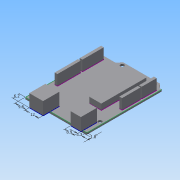
# Autodesk Inventor part: arduino_uno
Saved by Autodesk Inventor 2015 (Build 190159000, 159)
## iProperties
Created: 2016-01-04
Part Number: arduino_uno
Material: Generic
Document SubType Name: Modeling
Designer: JoshuaYuan
Density: 1 g/cm^3
Appearance: Default
Author: JoshuaYuan
Autodesk Inventor part; units mm, degrees
ref_plane "YZ Plane" through (0, 0, 0) normal (1, 0, 0) x (0, 1, 0)
ref_plane "XZ Plane" through (0, 0, 0) normal (0, 1, 0) x (-1, 0, 0)
ref_plane "XY Plane" through (0, 0, 0) normal (0, 0, 1) x (1, 0, 0)
sketch "Sketch1" plane through (0, 0, 0) normal (0, 1, 0) x (-1, 0, 0)
  line L0 (53.3, 0) -> (0, 0)
  line L1 (0, 0) -> (0, -65)
  line L2 (0, -65) -> (2, -65)
  line L3 (2, -65) -> (5, -68.6)
  line L4 (5, -68.6) -> (37, -68.6)
  line L5 (37, -68.6) -> (40, -65)
  line L6 (40, -65) -> (52.46, -65)
  line L7 (52.46, -65) -> (53.3, -64.3)
  line L8 (53.3, -64.3) -> (53.3, 0)
  line L9 (63.96, 0) -> (-10.66, 0) projected
  line L10 (0, -82.32) -> (0, 13.72) projected
  circle A0 centre (50.3, -15.1) radius 1.6
  circle A1 centre (2.5, -14) radius 1.6
  circle A2 centre (35.1, -65.9) radius 1.6
  circle A3 centre (7.2, -65.9) radius 1.6
  dimension "d2" = 53.3
  dimension "d5" = 51.9
  dimension "d6" = 1.1
  dimension "d8" = 27.9
  dimension "d9" = 15.2
  dimension "d10" = 68.6
  dimension "d11" = 3.2
  dimension "d12" = 50.8
  dimension "d13" = 4.7
  dimension "d15" = 2.5
  dimension "d17" = 14
  dimension "d18" = 37
  dimension "d19" = 40
  dimension "d20" = 2
  dimension "d21" = 5
  dimension "d22" = 65
  constraints: 18 end point, 4 centre point, 3 equal radius, 3 perpendicular, 2 parallel, 2 point on line, 1 collinear, 1 horizontal
  measures "d2" distance of L0.end L0.start
  measures "d5" vertical distance of A1.centre A3.centre
  measures "d6" vertical distance of A1.centre A0.centre
  measures "d8" distance of A2.centre A3.centre
  measures "d9" horizontal distance of A0.centre A2.centre
  measures "d10" distance between parallel lines of L4 L0
  measures "d11" diameter of A0
  measures "d12" vertical distance of A2.centre A0.centre
  measures "d13" horizontal distance of A3.centre A1.centre
  measures "d15" distance from line of L1 A1.centre
  measures "d17" distance from line of A1.centre L0
  measures "d18" distance from line of L1 L4.end
  measures "d19" distance from line of L1 L5.end
  measures "d20" distance of L1.end L2.end
  measures "d21" distance from line of L1 L3.end
  measures "d22" distance between parallel lines of L2 L0
extrude "board" add sketch "Sketch1" along normal blind 1.6
sketch "Sketch2" plane through (0, 1.6, 0) normal (0, 1, 0) x (1, 0, 0)
  line L0 (-43.7, -6.2) -> (-31.7, -6.2)
  line L1 (-31.7, -6.2) -> (-31.7, 7.8481)
  line L2 (-31.7, 7.8481) -> (-43.7, 7.8481)
  line L3 (-43.7, 7.8481) -> (-43.7, -6.2)
  line L4 (-12.2, -1.8) -> (-3.3, -1.8)
  line L5 (-3.3, -1.8) -> (-3.3, 12.0502)
  line L6 (-3.3, 12.0502) -> (-12.2, 12.0502)
  line L7 (-12.2, 12.0502) -> (-12.2, -1.8)
  line L8 (-50.0547, 22.1848) -> (-47.7065, 22.1848)
  line L9 (-47.7065, 22.1848) -> (-47.7065, 42.392)
  line L10 (-47.7065, 42.392) -> (-50.0547, 42.392)
  line L11 (-50.0547, 42.392) -> (-50.0547, 22.1848)
  line L12 (-50.0547, 43.9369) -> (-47.7065, 43.9369)
  line L13 (-47.7065, 43.9369) -> (-47.7065, 62.4757)
  line L14 (-47.7065, 62.4757) -> (-50.0547, 62.4757)
  line L15 (-50.0547, 62.4757) -> (-50.0547, 43.9369)
  line L16 (-3.9549, 32.1957) -> (-1.6067, 32.1957)
  line L17 (-1.6067, 32.1957) -> (-1.6067, 48.2627)
  line L18 (-1.6067, 48.2627) -> (-3.9549, 48.2627)
  line L19 (-3.9549, 48.2627) -> (-3.9549, 32.1957)
  line L20 (-3.9549, 49.2514) -> (-1.6067, 49.2514)
  line L21 (-1.6067, 49.2514) -> (-1.6067, 62.2285)
  line L22 (-1.6067, 62.2285) -> (-3.9549, 62.2285)
  line L23 (-3.9549, 62.2285) -> (-3.9549, 49.2514)
  line L24 (-53.3, 64.3) -> (-53.3, 0) projected
  line L25 (0, 0) -> (0, 65) projected
  line L26 (-53.3, 0) -> (0, 0) projected
  line L27 (-20.8879, 23.0716) -> (-10.5062, 23.0716)
  line L28 (-10.5062, 23.0716) -> (-10.5062, 62.2285)
  line L29 (-10.5062, 62.2285) -> (-20.8879, 62.2285)
  line L30 (-20.8879, 62.2285) -> (-20.8879, 23.0716)
  dimension "d25" = 9.6
  dimension "d26" = 12
  dimension "d27" = 3.3
  dimension "d28" = 8.9
  dimension "d29" = 1.8
  dimension "d30" = 6.2
  constraints: 56 end point, 15 parallel, 7 horizontal, 7 perpendicular, 4 point on line
  measures "d25" distance between parallel lines of L24 L3
  measures "d26" distance of L0.start L0.end
  measures "d27" distance between parallel lines of L25 L5
  measures "d28" distance of L4.start L4.end
  measures "d29" distance between parallel lines of L26 L4
  measures "d30" distance between parallel lines of L26 L0
extrude "Extrusion2" add sketch "Sketch2" along normal blind 10.9 contours L3 L26 L1 L0 | L3 L2 L1 L26 | L7 L26 L5 L4 | L7 L6 L5 L26
extrude "Extrusion3" add sketch "Sketch2" along normal blind 5 contours L30 L29 L28 L27
extrude "Extrusion4" add sketch "Sketch2" along normal blind 9 contours L11 L10 L9 L8 | L15 L14 L13 L12 | L19 L18 L17 L16 | L23 L22 L21 L20
body "Solid1"
